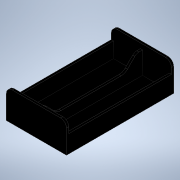
# Autodesk Inventor part: porta pila
Saved by Autodesk Inventor 2020 (Build 240168000, 168)
## iProperties
Created: 2022-05-20
Part Number: porta pila
Material: Generic
Document SubType Name: Modeling
Designer: juanc
Density: 1 g/cm^3
Appearance: Default
Author: juanc
Autodesk Inventor part; units mm, degrees
ref_plane "YZ Plane" through (0, 0, 0) normal (1, 0, 0) x (0, 1, 0)
ref_plane "XZ Plane" through (0, 0, 0) normal (0, 1, 0) x (-1, 0, 0)
ref_plane "XY Plane" through (0, 0, 0) normal (0, 0, 1) x (1, 0, 0)
sketch "Sketch1" plane through (0, 0, 0) normal (0, 0, 1) x (1, 0, 0)
  line L0 (0, 0) -> (41, 0)
  line L1 (41, 0) -> (41, 20)
  line L2 (41, 20) -> (0, 20)
  line L3 (0, 20) -> (0, 0)
  dimension "d0" = 41
  dimension "d1" = 20
  constraints: 8 end point, 2 parallel, 1 horizontal, 1 perpendicular
  measures "d0" distance of L2.end L1.end
  measures "d1" distance of L1.end L0.end
extrude "Extrusion1" add sketch "Sketch1" along normal blind 1.5
fillet "Fillet1" radius 4 2 edges at (41, 20, 0.75) (0, 20, 0.75)
sketch "Sketch3" plane through (0, 0, 0) normal (0, 0, -1) x (-1, 0, 0)
  line L0 (0, 0) -> (-41, 0) projected
  line L1 (-41, 0) -> (-39.5, 0)
  line L2 (-39.5, 0) -> (-39.5, 12)
  line L3 (-39.5, 12) -> (-41, 12)
  line L4 (-41, 12) -> (-41, 0)
  dimension "d5" = 1.5
  dimension "d6" = 12
  constraints: 8 end point, 2 parallel, 1 horizontal, 1 perpendicular
  measures "d5" distance of L3.end L2.end
  measures "d6" distance of L2.end L1.end
extrude "Extrusion2" add sketch "Sketch3" along normal blind 70
sketch "Sketch4" plane through (0, 0, 0) normal (0, 0, -1) x (-1, 0, 0)
  line L0 (0, 0) -> (-39.5, 0) projected
  line L1 (0, 0) -> (-1.5, 0)
  line L2 (-1.5, 0) -> (-1.5, 12)
  line L3 (-1.5, 12) -> (0, 12)
  line L4 (0, 12) -> (0, 0)
  dimension "d9" = 1.5
  dimension "d10" = 12
  constraints: 8 end point, 2 parallel, 1 horizontal, 1 perpendicular
  measures "d9" distance of L2.end L3.end
  measures "d10" distance of L1.end L2.end
extrude "Extrusion3" add sketch "Sketch4" along normal blind 70
sketch "Sketch5" plane through (0, 0, -70) normal (0, 0, -1) x (-1, 0, 0)
  line L0 (-41, 0) -> (-41, 16) projected
  line L1 (-41, 0) -> (0, 0)
  line L2 (0, 0) -> (0, 20)
  line L3 (0, 20) -> (-41, 20)
  line L4 (-41, 20) -> (-41, 0)
  constraints: 8 end point, 2 parallel, 1 horizontal, 1 perpendicular
extrude "Extrusion4" add sketch "Sketch5" along normal blind 1.5
fillet "Fillet2" radius 4 2 edges at (0, 20, -70.75) (41, 20, -70.75)
sketch "Sketch6" plane through (0, 0, 1.5) normal (0, -1, 0) x (1, 0, 0)
  line L0 (4, -73) -> (0, -73) projected
  line L1 (41, 0) -> (41, -1.5) projected
  line L2 (0, -73) -> (41, -73)
  line L3 (41, -73) -> (41, 0)
  line L4 (41, 0) -> (0, 0)
  line L5 (0, 0) -> (0, -73)
  point P0 (0, -1.5)
  constraints: 8 end point, 2 parallel, 1 horizontal, 1 perpendicular
extrude "Extrusion5" add sketch "Sketch6" against normal blind 1.5
ref_plane "Work Plane1" through (20.5, 0, 1.5) normal (1, 0, 0) x (0, 0, -1)
sketch "Sketch9" plane through (20.5, 0, 1.5) normal (1, 0, 0) x (0, 0, -1)
  line L0 (71.5, 1.5) -> (59.5, 1.5)
  line L1 (59.5, 1.5) -> (59.5, 16.5)
  line L2 (59.5, 16.5) -> (71.5, 16.5)
  line L3 (71.5, 16.5) -> (71.5, 1.5)
  point P0 (1.5, 0)
  dimension "d25" = 12
  dimension "d26" = 15
  constraints: 8 end point, 2 parallel, 1 horizontal, 1 perpendicular
  measures "d25" distance of L1.end L2.end
  measures "d26" distance of L0.end L1.end
extrude "Extrusion6" add sketch "Sketch9" along normal mid plane 1.5
chamfer "Chamfer1" distance 8 angle 45 1 edges at (20.5, 16.5, -58)
fillet "Fillet3" radius 4 1 edges at (20.5, 16.5, -66)
sketch "Sketch10" plane through (20.5, 0, 1.5) normal (1, 0, 0) x (0, 0, -1)
  line L0 (1.5, 1.5) -> (13.5, 1.5)
  line L1 (13.5, 1.5) -> (13.5, 16.5)
  line L2 (13.5, 16.5) -> (1.5, 16.5)
  line L3 (1.5, 16.5) -> (1.5, 1.5)
  point P0 (1.5, 0)
  dimension "d27" = 12
  dimension "d28" = 15
  constraints: 8 end point, 2 parallel, 1 horizontal, 1 perpendicular
  measures "d27" distance of L2.end L1.end
  measures "d28" distance of L1.end L0.end
extrude "Extrusion7" add sketch "Sketch10" along normal mid plane 1.5
chamfer "Chamfer2" distance 8 angle 45 1 edges at (20.5, 16.5, -12)
fillet "Fillet4" radius 4 1 edges at (20.5, 16.5, -4)
sketch "Sketch11" plane through (21.25, 1.5, -12) normal (0, 0, -1) x (-1, 0, 0)
  line L0 (1.5, 7) -> (1.5, 0) projected
  line L1 (0, 0) -> (1.5, 0)
  line L2 (1.5, 0) -> (1.5, 7)
  line L3 (1.5, 7) -> (0, 7)
  line L4 (0, 7) -> (0, 0)
  point P0 (21.25, -1.5)
  constraints: 8 end point, 2 parallel, 1 horizontal, 1 perpendicular
extrude "Extrusion8" add sketch "Sketch11" along normal blind 50
fillet "Fillet5" radius 6 2 edges at (20.5, 8.5, -58) (20.5, 8.5, -12)
body "Solid1"
